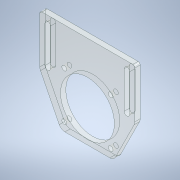
# Autodesk Inventor part: 103.006.01_Dosiereinheit_Rahmenaufnahme
Saved by Autodesk Inventor 2021 (Build 250183000, 183)
## iProperties
Created: 2020-11-24
Part Number: 103.006.01_Dosiereinheit_Rahmenaufnahme
Material: Generic
Document SubType Name: Modeling
Designer: Alexander Fritzsche
Density: 1 g/cm^3
Appearance: Default
Author: Alexander Fritzsche
Autodesk Inventor part; units mm, degrees
ref_plane "YZ Plane" through (0, 0, 0) normal (1, 0, 0) x (0, 1, 0)
ref_plane "XZ Plane" through (0, 0, 0) normal (0, 1, 0) x (-1, 0, 0)
ref_plane "XY Plane" through (0, 0, 0) normal (0, 0, 1) x (1, 0, 0)
sketch "Sketch1" plane through (0, 0, 0) normal (0, 0, 1) x (1, 0, 0)
  line L0 (-45, 43.75) -> (45, 43.75)
  line L1 (45, 43.75) -> (45, -3.75)
  line L2 (45, -3.75) -> (25, -43.75)
  line L3 (25, -43.75) -> (-25, -43.75)
  line L4 (-25, -43.75) -> (-45, -3.75)
  line L5 (-45, -3.75) -> (-45, 43.75)
  line L6 (0, 53.6312) -> (0, 0)
  line L7 (0, 0) -> (107.3954, 0)
  line L8 (-37.5, 36.25) -> (-37.5, 1.25) construction
  line L9 (-40.1, 36.25) -> (-40.1, 1.25)
  line L10 (-34.9, 1.25) -> (-34.9, 36.25)
  arc A0 (-34.9, 36.25) -> (-40.1, 36.25) centre (-37.5, 36.25) ccw
  arc A1 (-40.1, 1.25) -> (-34.9, 1.25) centre (-37.5, 1.25) ccw
  line L11 (37.5, 36.25) -> (37.5, 1.25) construction
  line L12 (34.9, 36.25) -> (34.9, 1.25)
  line L13 (40.1, 1.25) -> (40.1, 36.25)
  arc A2 (40.1, 36.25) -> (34.9, 36.25) centre (37.5, 36.25) ccw
  arc A3 (34.9, 1.25) -> (40.1, 1.25) centre (37.5, 1.25) ccw
  line L14 (-37.5, 36.25) -> (167.5, 36.25) construction
  point P0 (-37.5, 18.75)
  point P1 (37.5, 18.75)
  dimension "d1" = 87.5
  dimension "d2" = 47.5
  dimension "d3" = 2.6
  dimension "d4" = 35
  dimension "d5" = 7.5
  dimension "d6" = 7.5
  dimension "d7" = 75
  dimension "d9" = 20
  dimension "d40" = 7.5
  dimension "d41" = 5.2
  dimension "d42" = 5.2
  dimension "d45" = 42.5
  constraints: 34 end point, 8 point on circle, 8 tangent, 6 parallel, 4 centre point, 2 horizontal, 2 midpoint, 2 perpendicular, 2 vertical, 1 equal radius, 1 point on line, 3 other
  measures "d1" distance between parallel lines of L3 L0
  measures "d2" distance of L0.end L1.end
  measures "d3" radius of A1
  measures "d4" distance of L8.start L8.end
  measures "d5" distance from line of L0 L8.start
  measures "d6" distance from line of L5 L8.start
  measures "d7" distance between parallel lines of L11 L8
  measures "d9" distance from line of L3.end L5
  measures "d40" distance between parallel lines of L1 L11
  measures "d41" distance between parallel lines of L12 L13
  measures "d42" distance between parallel lines of L9 L10
  measures "d45" distance from line of L8.end L0
extrude "Extrusion1" add sketch "Sketch1" along normal blind 5 contours L0 L6 L7 A3 L1 L2 L3 L4 L5 | L0 L1 L7 A3 L13 A2 L12 L6
fillet "Fillet1" radius 2 2 edges at (-45, 43.75, 2.5) (45, 43.75, 2.5)
sketch "Sketch2" plane through (0, 0, 5) normal (0, 0, 1) x (1, 0, 0)
  line L0 (0.1, -13.75) -> (0.1, 26.1696) construction
  line L1 (-34.9, 36.25) -> (-34.9, 1.25) projected
  line L2 (-25, -43.75) -> (25, -43.75) projected
  point P0 (0, 0)
  point P1 (-23.7639, -52.5)
  point P2 (23.7639, -52.5)
  dimension "d23" = 35
  dimension "d24" = 30
  constraints: 2 end point, 1 vertical, 1 other
  measures "d23" distance between parallel lines of L0 L1
hole "Hole1" at (0.1, -13.75, 5) direction (0, 0, -1) diameter 51 end through all
sketch "Sketch3" plane through (0, 0, 5) normal (0, 0, 1) x (1, 0, 0)
  circle A0 centre (0.1, -13.75) radius 25.5 projected
  point P0 (0, 0)
  point P1 (-21.9, 8.25)
  dimension "d32" = 22
  dimension "d33" = 22
  measures "d32" horizontal distance of A0.centre point (-21.9, 8.25)
  measures "d33" horizontal distance of A0.centre point (-21.9, 8.25)
hole "Hole2" at (-21.9, 8.25, 5) direction (0, 0, -1) diameter 4.5 end through all
pattern_linear "Rectangular Pattern2" count 2 spacing 44 along (1, 0, 0) count 2 spacing 44 along (0, -1, 0) of "Hole2"
fillet "Rundung2" radius 6 4 edges at (45, -3.75, 2.5) (25, -43.75, 2.5) (-25, -43.75, 2.5) (-45, -3.75, 2.5)
equation "\"d6\" = d5"
equation "\"d33\" = d32"
equation "\"d36\" = 2 * d32"
equation "\"d39\" = 2 * d32"
body "Solid1"
